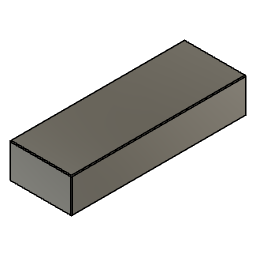
Staedtler rubber_ (Autodesk Fusion 360 design; units mm, degrees)
Autodesk Fusion 360 part; units mm, degrees
sketch "Sketch1" plane through (0, 0, 0) normal (0, 0, 1) x (1, 0, 0)
  line L0 (0, 0) -> (-23, 0)
  line L1 (-23, 0) -> (-23, 65)
  line L2 (-23, 65) -> (0, 65)
  line L3 (0, 65) -> (0, 0)
  dimension "d1" = 23
  dimension "d2" = 65
  constraint horizontal L0
  constraint vertical L1
  constraint horizontal L2
  constraint vertical L3
  constraint coincident L0.start L3.end
  measures "d1" distance of L0.start L0.end
  measures "d2" distance of L0.start L2.end
extrude "Extrude1" add sketch "Sketch1" along normal blind 13
fillet "Fillet1" radius 0.3 12 edges at (0, 32.5, 13) (0, 32.5, 0) (-23, 32.5, 13) (-23, 32.5, 0) (-11.5, 0, 13) (-23, 0, 6.5) (-11.5, 0, 0) (0, 0, 6.5) (-11.5, 65, 13) (-11.5, 65, 0) (0, 65, 6.5) (-23, 65, 6.5)
